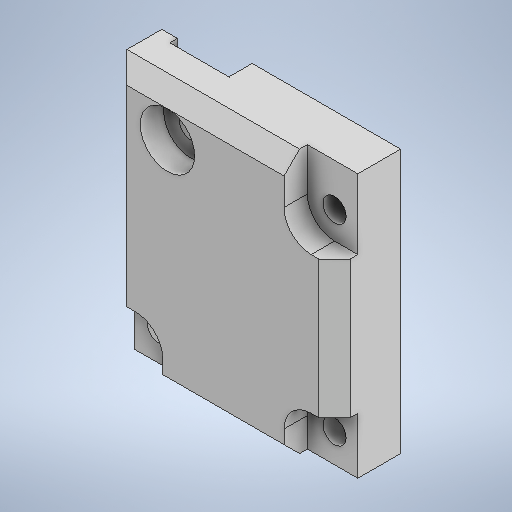
# Autodesk Inventor part: LatchCover
Saved by Autodesk Inventor 2025.1 (Build 291241000, 241)
## iProperties
Created: 2026-05-10
Part Number: LatchCover
Material: Generic
Document SubType Name: Modeling
Designer: User
Density: 1 g/cm^3
Appearance: Default
Author: User
## iProperties of the stored document LatchCover_3DPrint.ipt
Created: 2026-05-12
Part Number: LatchCover_3DPrint
Material: Generic
Document SubType Name: Modeling
Designer: User
Density: 1 g/cm^3
Appearance: Default
Author: User
Autodesk Inventor part; units mm, degrees
ref_plane "YZ Plane" through (0, 0, 0) normal (1, 0, 0) x (0, 1, 0)
ref_plane "XZ Plane" through (0, 0, 0) normal (0, 1, 0) x (-1, 0, 0)
sketch "Sketch1" plane through (0, 0, 0) normal (0, 0, 1) x (1, 0, 0)
  circle A0 centre (13.604, -26.2353) radius 1.6 projected
  line L0 (18.604, -44.1888) -> (15.604, -44.1888) projected
  line L1 (15.604, -44.1888) -> (15.604, -37.1888) projected
  line L2 (15.604, -37.1888) -> (18.604, -37.1888) projected
  line L3 (18.604, -26.2353) -> (18.604, -37.1888) projected
  arc A1 (18.604, -26.2353) -> (8.604, -26.2353) centre (13.604, -26.2353) ccw projected
  line L4 (8.604, -26.2353) -> (8.604, -45.6888) projected
  line L5 (9.104, -46.1888) -> (8.604, -45.6888) projected
  line L6 (9.104, -46.1888) -> (12.604, -46.1888) projected
  line L7 (13.104, -46.6888) -> (12.604, -46.1888) projected
  line L8 (13.104, -46.6888) -> (13.104, -55.1706) projected
  line L9 (12.604, -55.6706) -> (13.104, -55.1706) projected
  line L10 (12.604, -55.6706) -> (3.2048, -55.6706) projected
  line L11 (3.2048, -55.6706) -> (3.2048, -62.5334) projected
  line L12 (3.2048, -62.5334) -> (8.604, -62.5334) projected
  line L13 (8.604, -62.5334) -> (8.604, -81.1802) projected
  line L14 (8.604, -81.1802) -> (9.604, -81.1802) projected
  line L15 (9.604, -62.5334) -> (9.604, -81.1802) projected
  line L16 (9.604, -62.5334) -> (17.604, -62.5334) projected
  line L17 (17.604, -81.1802) -> (17.604, -62.5334) projected
  line L18 (17.604, -81.1802) -> (18.604, -81.1802) projected
  line L19 (18.604, -44.1888) -> (18.604, -81.1802) projected
  line L20 (19.104, -37.6888) -> (16.104, -37.6888)
  line L21 (16.104, -37.6888) -> (16.104, -43.6888)
  line L22 (16.104, -43.6888) -> (19.104, -43.6888)
  line L23 (19.104, -43.6888) -> (19.104, -81.6802)
  line L24 (19.104, -81.6802) -> (17.104, -81.6802)
  line L25 (17.104, -81.6802) -> (17.104, -63.0334)
  line L26 (17.104, -63.0334) -> (10.104, -63.0334)
  line L27 (10.104, -63.0334) -> (10.104, -81.6802)
  line L28 (10.104, -81.6802) -> (8.104, -81.6802)
  line L29 (8.104, -81.6802) -> (8.104, -63.0334)
  line L30 (8.104, -63.0334) -> (2.7048, -63.0334)
  line L31 (2.7048, -63.0334) -> (2.7048, -55.1706)
  line L32 (2.7048, -55.1706) -> (12.3969, -55.1706)
  line L33 (12.3969, -55.1706) -> (12.604, -54.9635)
  line L34 (12.604, -54.9635) -> (12.604, -46.8959)
  line L35 (12.604, -46.8959) -> (12.3969, -46.6888)
  line L36 (12.3969, -46.6888) -> (8.8969, -46.6888)
  line L37 (8.8969, -46.6888) -> (8.104, -45.8959)
  line L38 (8.104, -45.8959) -> (8.104, -26.2353)
  arc A2 (19.104, -26.2353) -> (8.104, -26.2353) centre (13.604, -26.2353) ccw
  line L39 (19.104, -26.2353) -> (19.104, -37.6888)
  line L40 (30.104, -37.6888) -> (30.104, -43.6888)
  line L41 (19.604, -38.1888) -> (16.604, -38.1888)
  line L42 (16.604, -38.1888) -> (16.604, -43.1888)
  line L43 (16.604, -43.1888) -> (19.604, -43.1888)
  line L44 (19.604, -43.1888) -> (19.604, -82.1802)
  line L45 (19.604, -82.1802) -> (16.604, -82.1802)
  line L46 (16.604, -82.1802) -> (16.604, -63.5334)
  line L47 (16.604, -63.5334) -> (10.604, -63.5334)
  line L48 (10.604, -63.5334) -> (10.604, -82.1802)
  line L49 (10.604, -82.1802) -> (7.604, -82.1802)
  line L50 (7.604, -82.1802) -> (7.604, -63.5334)
  line L51 (7.604, -63.5334) -> (2.2048, -63.5334)
  line L52 (2.2048, -63.5334) -> (2.2048, -54.6706)
  line L53 (2.2048, -54.6706) -> (12.104, -54.6706)
  line L54 (12.104, -54.6706) -> (12.104, -47.1888)
  line L55 (12.104, -47.1888) -> (8.6898, -47.1888)
  line L56 (8.6898, -47.1888) -> (7.604, -46.103)
  line L57 (7.604, -46.103) -> (7.604, -26.2353)
  arc A3 (19.604, -26.2353) -> (7.604, -26.2353) centre (13.604, -26.2353) ccw
  line L58 (19.604, -26.2353) -> (19.604, -38.1888)
  circle A4 centre (9.4965, -50.9297) radius 1.5 projected
  line L59 (30.104, -37.6888) -> (35.104, -37.6888)
  line L60 (13.604, -20.7353) -> (35.104, -20.7353)
  line L61 (13.604, -20.7353) -> (35.104, -20.7353) construction
  line L62 (12.104, -54.6706) -> (35.104, -54.6706)
  line L63 (35.104, -54.6706) -> (35.104, -20.7353)
  line L64 (6.389, 0.2) -> (6.389, -55.4706) projected
  line L65 (19.604, -54.6706) -> (25.604, -54.6706)
  line L66 (35.104, -20.7353) -> (32.104, -20.7353)
  line L67 (32.104, -24.7353) -> (32.104, -52.4297)
  line L68 (9.4965, -50.9297) -> (32.104, -50.9297)
  circle A5 centre (32.104, -26.2353) radius 1.5
  circle A6 centre (32.104, -50.9297) radius 1.5
  line L69 (25.604, -54.6706) -> (23.3357, -43.6888)
  line L70 (16.104, -37.6888) -> (19.604, -37.6888)
  line L71 (22.0964, -37.6888) -> (30.104, -37.6888)
  line L72 (30.104, -43.6888) -> (23.3357, -43.6888)
  line L73 (19.604, -43.6888) -> (19.104, -43.6888)
  line L74 (22.0964, -37.6888) -> (19.4799, -25.0216)
  line L75 (18.5946, -20.7353) -> (18.0297, -18.0002)
  line L76 (13.604, -26.2353) -> (19.7306, -26.2353)
  line L77 (30.604, -26.2353) -> (32.104, -26.2353)
  point P0 (0, 0)
  point P1 (16.0019, -20.7353)
  dimension "d10" = 3
  dimension "d0" = 0.5
  dimension "d2" = 14
  dimension "d3" = 0.5
  dimension "d4" = 5
  dimension "d5" = 0
  dimension "d6" = 3.1842
  dimension "d7" = 6
  dimension "d8" = 3
  dimension "d9" = 3
  constraints: 114 end point, 10 point on line, 8 point on circle, 7 perpendicular, 3 centre point, 3 horizontal, 3 tangent, 2 coincident, 2 parallel, 1 collinear, 1 vertical, 1 vertical alignment, 40 other
  measures "d0" distance between parallel lines of L2 L20
  measures "d2" distance of L20.end L40.start
  measures "d3" distance between parallel lines of L39 L58
  measures "d4" distance of L40.start L59.end
  measures "d5" distance between parallel lines of L60 L61
  measures "d6" distance between parallel lines of L11 L64
  measures "d7" distance of L65.start L65.end
  measures "d8" distance of L61.end L66.end
  measures "d9" diameter of A5
extrude "Extrusion1" add sketch "Sketch1" along normal blind 7 contours L69 L72 L40 L59 L67 A6 L68 | L68 A6 L67 L59 L63 L62 L69 | L60 L63 L59 L71 L74 A3
sketch "Sketch2" plane through (0, 0, 7) normal (0, 0, 1) x (1, 0, 0)
  line L0 (25.604, -54.6706) -> (35.104, -54.6706) projected
  line L1 (35.104, -54.6706) -> (35.104, -20.7353) projected
  line L2 (35.104, -20.7353) -> (16.0019, -20.7353) projected
  arc A0 (19.4799, -25.0216) -> (16.0019, -20.7353) centre (13.604, -26.2353) ccw projected
  line L3 (19.4799, -25.0216) -> (22.0964, -37.6888) projected
  line L4 (22.0964, -37.6888) -> (30.104, -37.6888) projected
  line L5 (30.104, -37.6888) -> (30.104, -43.6888) projected
  line L6 (30.104, -43.6888) -> (23.3357, -43.6888) projected
  line L7 (23.3357, -43.6888) -> (25.604, -54.6706) projected
  circle A1 centre (32.104, -50.9297) radius 1.5 projected
  circle A2 centre (32.104, -26.2353) radius 1.5 projected
  circle A3 centre (13.604, -26.2353) radius 1.5 projected
  circle A4 centre (9.4965, -50.9297) radius 1.5 projected
  line L8 (6.389, 0.2) -> (6.389, -55.4706) projected
  line L9 (35.104, -20.7353) -> (6.389, -20.7353)
  line L10 (25.604, -54.6706) -> (35.104, -54.6706) projected
  line L11 (35.104, -54.6706) -> (6.389, -54.6706)
  point P0 (0, 0)
  constraints: 4 end point, 3 point on line, 1 perpendicular
extrude "Extrusion2" add sketch "Sketch2" along normal blind 1.5
sketch "Sketch3" plane through (0, 0, 7) normal (0, 0, -1) x (-1, 0, 0)
  line L0 (-15.604, -37.1888) -> (-15.604, -44.1888) projected
  line L1 (-18.604, -37.1888) -> (-15.604, -37.1888) projected
  line L2 (-15.604, -44.1888) -> (-18.604, -44.1888) projected
  line L3 (-19.4799, -25.0216) -> (-22.0964, -37.6888) projected
  arc A0 (-16.0019, -20.7353) -> (-19.4799, -25.0216) centre (-13.604, -26.2353) ccw projected
  line L4 (-16.0019, -20.7353) -> (-6.389, -20.7353) projected
  line L5 (-6.389, -78.3802) -> (-6.389, 0.2) projected
  line L6 (-6.389, -54.6706) -> (-25.604, -54.6706) projected
  line L7 (-23.3357, -43.6888) -> (-25.604, -54.6706) projected
  line L8 (-15.604, -37.1888) -> (-21.9931, -37.1888)
  line L9 (-15.604, -44.1888) -> (-23.4389, -44.1888)
  circle A1 centre (-13.604, -26.2353) radius 1.5 projected
  circle A2 centre (-9.4965, -50.9297) radius 1.5 projected
  point P0 (0, 0)
  constraints: 4 end point, 3 point on line, 1 horizontal
extrude "Extrusion3" add sketch "Sketch3" along normal blind 4
sketch "Sketch4" plane through (0, 0, 8.5) normal (0, 0, 1) x (1, 0, 0)
  circle A0 centre (32.104, -26.2353) radius 1.5 projected
  circle A1 centre (13.604, -26.2353) radius 1.5 projected
  circle A2 centre (9.4965, -50.9297) radius 1.5 projected
  circle A3 centre (32.104, -50.9297) radius 1.5 projected
  circle A4 centre (32.104, -26.2353) radius 3.5
  circle A5 centre (13.604, -26.2353) radius 3.5
  circle A6 centre (32.104, -50.9297) radius 3.5
  circle A7 centre (9.4965, -50.9297) radius 3.5
  line L0 (35.104, -54.6706) -> (35.104, -20.7353) projected
  line L1 (6.389, -54.6706) -> (35.104, -54.6706) projected
  line L2 (6.5058, -78.3802) -> (6.5058, 0.2)
  line L3 (9.4965, -47.4297) -> (6.5058, -47.4297)
  line L4 (12.9965, -50.9297) -> (12.9965, -54.6706)
  line L5 (28.604, -50.9297) -> (28.604, -54.6706)
  line L6 (32.104, -47.4297) -> (35.104, -47.4297)
  line L7 (35.104, -29.7353) -> (32.104, -29.7353)
  line L8 (28.604, -26.2353) -> (28.604, -20.7353)
  line L9 (35.104, -20.7353) -> (16.0019, -20.7353) projected
  point P0 (0, 0)
  point P1 (6.5058, -54.6706)
  dimension "d17" = 7
  dimension "d18" = 7
  dimension "d19" = 7
  dimension "d20" = 7
  constraints: 14 end point, 8 point on line, 6 point on circle, 4 centre point, 4 coincident, 4 perpendicular, 3 tangent, 1 horizontal, 1 vertical, 2 other
  measures "d17" diameter of A4
  measures "d18" diameter of A5
  measures "d19" diameter of A6
  measures "d20" diameter of A7
extrude "Extrusion4" cut sketch "Sketch4" against normal blind 3 contours A4 L0 | L8 L9 L0 A4 | A4 L0 L7 | A5 | A6 L0 | L6 L0 A6 | A6 L0 L1 L5 | A7 L2 | L4 L1 L2 A7 | A7 L2 L3 picked at (34.604, -26.2353) picked at (34.604, -50.9297) picked at (7.0027, -50.9297)
sketch "Sketch5" plane through (0, 0, 8.5) normal (0, 0, 1) x (1, 0, 0)
  line L0 (6.5058, -54.6706) -> (6.5058, -47.4297) projected
  line L1 (6.389, -54.6706) -> (6.5058, -54.6706) projected
  line L2 (6.389, -20.7353) -> (6.389, -54.6706) projected
  line L3 (6.5058, -54.6706) -> (6.1522, -54.6706)
  line L4 (6.1522, -54.6706) -> (6.1522, -47.4297)
  line L5 (6.1522, -47.4297) -> (6.5058, -47.4297)
  line L6 (6.5058, -47.4297) -> (6.5058, -54.6706)
  point P0 (0, 0)
  constraints: 8 end point, 2 parallel, 1 horizontal, 1 perpendicular
extrude "Extrusion5" cut sketch "Sketch5" against normal up to surface (3 mm away)
chamfer "Chamfer1" distance 2 angle 45 4 edges at (6.389, -34.0825, 8.5) (35.104, -38.5825, 8.5) (17.4965, -20.7353, 8.5) (20.8002, -54.6706, 8.5)
sketch "Sketch6" plane through (0, 0, 3) normal (0, 0, -1) x (-1, 0, 0)
  line L0 (-6.389, -54.6706) -> (-6.389, -20.7353) projected
  line L1 (-6.389, -55.1706) -> (-12.3969, -55.1706) projected
  line L2 (-12.604, -54.9635) -> (-12.3969, -55.1706) projected
  line L3 (-12.604, -46.8959) -> (-12.604, -54.9635) projected
  line L4 (-12.3969, -46.6888) -> (-12.604, -46.8959) projected
  line L5 (-8.404, -46.6888) -> (-12.3969, -46.6888) projected
  line L6 (-8.404, -20.7353) -> (-8.404, -46.6888) projected
  line L7 (-8.404, 3) -> (-8.404, -20.7353) projected
  line L8 (3.1786, 3) -> (-8.404, 3) projected
  line L9 (3.1786, 0.2) -> (3.1786, 3) projected
  line L10 (3.1786, 0.2) -> (-6.389, 0.2) projected
  line L11 (-6.389, 0.2) -> (-6.389, -55.1706) projected
  circle A0 centre (-9.4965, -50.9297) radius 1.5 projected
  line L12 (-6.389, -20.7353) -> (-16.0019, -20.7353) projected
  line L13 (-25.604, -54.6706) -> (-6.389, -54.6706) projected
  point P0 (0, 0)
  point P1 (-12.604, -54.6706)
ref_plane "Work Plane1" through (-23.745, -60.7506, 2.0147) normal (0, 0, 1) x (1, 0, 0)
extrude "Extrusion6" add sketch "Sketch6" along normal up to surface (0.9853 mm away) contours L13 L3 L4 L5 L6 L12 L0
body "Solid1"
